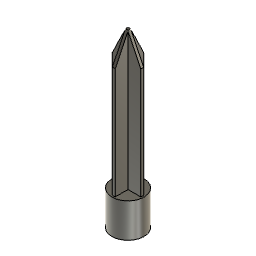
Target Ghost Lights Ground Stakes (Autodesk Fusion 360 design; units mm, degrees)
Autodesk Fusion 360 part; units mm, degrees
sketch "Sketch1" plane through (0, 0, 0) normal (0, 0, 1) x (1, 0, 0)
  circle A0 centre (0, 0) radius 11.25
  dimension "d1" = 22.5
  constraint coincident A0.centre origin
  measures "d1" diameter of A0
extrude "Extrude1" add sketch "Sketch1" along normal blind 21 makes body 1
sketch "Sketch2" plane through (0, 0, 0) normal (0, 0, 1) x (1, 0, 0)
  line L0 (-10, 1) -> (10, 1)
  line L1 (10, 1) -> (10, -1)
  line L2 (10, -1) -> (-10, -1)
  line L3 (-10, -1) -> (-10, 1)
  constraint horizontal L0
  constraint vertical L1
  constraint horizontal L2
  constraint vertical L3
extrude "Extrude2" add sketch "Sketch2" along normal blind 121 separate body makes body 2
sketch "Sketch3" plane through (0, 0, 0) normal (0, 0, 1) x (1, 0, 0)
  line L0 (-1, 10) -> (1, 10)
  line L1 (1, 10) -> (1, -10)
  line L2 (1, -10) -> (-1, -10)
  line L3 (-1, -10) -> (-1, 10)
  constraint horizontal L0
  constraint vertical L1
  constraint horizontal L2
  constraint vertical L3
extrude "Extrude3" add sketch "Sketch3" along normal blind 121 separate body makes body 3
sketch "Sketch5" plane through (0, 0, 0) normal (0, 1, 0) x (1, 0, 0)
  line L0 (0, -123) -> (11, -123)
  line L1 (11, -123) -> (11, -100)
  line L2 (11, -100) -> (1, -121)
  line L3 (1, -121) -> (0, -121)
  line L4 (0, -121) -> (0, -123)
  constraint horizontal L0
  constraint perpendicular L0 L1
  constraint perpendicular L1 L3
  constraint perpendicular L3 L4
revolve "Revolve1" cut sketch "Sketch5" angle 360 about axis through (0, 0, 1.75) along (0, 0, 1) bodies 2 3
sketch "Sketch6" plane through (0, 0, 0) normal (0, 0, 1) x (1, 0, 0)
  circle A0 centre (0, 0) radius 7
  dimension "d9" = 14
  constraint coincident A0.centre origin
  measures "d9" diameter of A0
extrude "Extrude4" add 1 faces at (1.0392, -6.3884, 21) along direction (0, 0, 1) blind 3 on bodies 1 bodies 1 2 3
extrude "Extrude5" cut sketch "Sketch6" along normal blind 21 bodies 1
